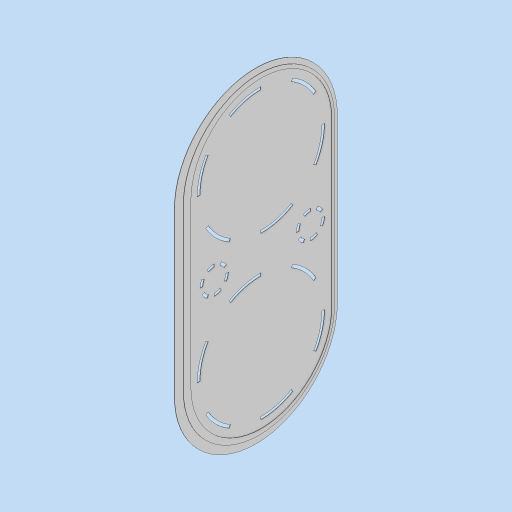
# Autodesk Inventor part: Sticker4
Saved by Autodesk Inventor 2024 (Build 280153000, 153)
## iProperties
Created: 2025-01-25
Part Number: Sticker4
Material: Generic
Document SubType Name: Modeling
Designer: Dmitry
Density: 1 g/cm^3
Appearance: Default
Author: Dmitry
Autodesk Inventor part; units mm, degrees
(part 1 of 2)
ref_plane "YZ Plane" through (0, 0, 0) normal (1, 0, 0) x (0, 1, 0)
ref_plane "XZ Plane" through (0, 0, 0) normal (0, 1, 0) x (-1, 0, 0)
ref_plane "XY Plane" through (0, 0, 0) normal (0, 0, 1) x (1, 0, 0)
sketch "Sketch1" plane through (0, 0, 0) normal (1, 0, 0) x (0, 1, 0)
  line L0 (-65.4167, -24.9139) -> (-65.4167, -26.1387)
  line L1 (-65.4167, -26.1387) -> (-65.6677, -29.8166)
  line L2 (-65.6677, -29.8166) -> (-66.4035, -34.5779)
  line L3 (-66.4035, -34.5779) -> (-67.5981, -39.175)
  line L4 (-67.5981, -39.175) -> (-69.2298, -43.5806)
  line L5 (-69.2298, -43.5806) -> (-71.2719, -47.7739)
  line L6 (-71.2719, -47.7739) -> (-73.7014, -51.7274)
  line L7 (-73.7014, -51.7274) -> (-76.4934, -55.4193)
  line L8 (-76.4934, -55.4193) -> (-79.6242, -58.8257)
  line L9 (-79.6242, -58.8257) -> (-83.0679, -61.921)
  line L10 (-83.0679, -61.921) -> (-86.8025, -64.6824)
  line L11 (-86.8025, -64.6824) -> (-90.8017, -67.0845)
  line L12 (-90.8017, -67.0845) -> (-95.0417, -69.1031)
  line L13 (-95.0417, -69.1031) -> (-99.4984, -70.717)
  line L14 (-99.4984, -70.717) -> (-104.1466, -71.8978)
  line L15 (-104.1466, -71.8978) -> (-108.9627, -72.6255)
  line L16 (-108.9627, -72.6255) -> (-112.682, -72.8737)
  line L17 (-112.682, -72.8737) -> (-113.9211, -72.8737)
  line L18 (-113.9211, -72.8737) -> (-115.1613, -72.8737)
  line L19 (-115.1613, -72.8737) -> (-118.8804, -72.6255)
  line L20 (-118.8804, -72.6255) -> (-123.6968, -71.8978)
  line L21 (-123.6968, -71.8978) -> (-128.345, -70.717)
  line L22 (-128.345, -70.717) -> (-132.8014, -69.1031)
  line L23 (-132.8014, -69.1031) -> (-137.0417, -67.0845)
  line L24 (-137.0417, -67.0845) -> (-141.0406, -64.6824)
  line L25 (-141.0406, -64.6824) -> (-144.7739, -61.921)
  line L26 (-144.7739, -61.921) -> (-148.2189, -58.8257)
  line L27 (-148.2189, -58.8257) -> (-151.3485, -55.4193)
  line L28 (-151.3485, -55.4193) -> (-154.1404, -51.7274)
  line L29 (-154.1404, -51.7274) -> (-156.5697, -47.7739)
  line L30 (-156.5697, -47.7739) -> (-158.6134, -43.5806)
  line L31 (-158.6134, -43.5806) -> (-160.2435, -39.175)
  line L32 (-160.2435, -39.175) -> (-161.4384, -34.5779)
  line L33 (-161.4384, -34.5779) -> (-162.1742, -29.8166)
  line L34 (-162.1742, -29.8166) -> (-162.4236, -26.1387)
  line L35 (-162.4236, -26.1387) -> (-162.4236, -24.9139)
  line L36 (-162.4236, -24.9139) -> (-162.4236, -23.6871)
  line L37 (-162.4236, -23.6871) -> (-162.1742, -20.0092)
  line L38 (-162.1742, -20.0092) -> (-161.4384, -15.2482)
  line L39 (-161.4384, -15.2482) -> (-160.2435, -10.6511)
  line L40 (-160.2435, -10.6511) -> (-158.6134, -6.2454)
  line L41 (-158.6134, -6.2454) -> (-156.5697, -2.0521)
  line L42 (-156.5697, -2.0521) -> (-154.1404, 1.9016)
  line L43 (-154.1404, 1.9016) -> (-151.3485, 5.5933)
  line L44 (-151.3485, 5.5933) -> (-148.2189, 8.9997)
  line L45 (-148.2189, 8.9997) -> (-144.7739, 12.0952)
  line L46 (-144.7739, 12.0952) -> (-141.0406, 14.8566)
  line L47 (-141.0406, 14.8566) -> (-137.0417, 17.2582)
  line L48 (-137.0417, 17.2582) -> (-132.8014, 19.2773)
  line L49 (-132.8014, 19.2773) -> (-128.345, 20.8909)
  line L50 (-128.345, 20.8909) -> (-123.6968, 22.072)
  line L51 (-123.6968, 22.072) -> (-118.8804, 22.7995)
  line L52 (-118.8804, 22.7995) -> (-115.1613, 23.0464)
  line L53 (-115.1613, 23.0464) -> (-113.9211, 23.0464)
  line L54 (-113.9211, 23.0464) -> (-112.682, 23.0464)
  line L55 (-112.682, 23.0464) -> (-108.9627, 22.7995)
  line L56 (-108.9627, 22.7995) -> (-104.1466, 22.072)
  line L57 (-104.1466, 22.072) -> (-99.4984, 20.8909)
  line L58 (-99.4984, 20.8909) -> (-95.0417, 19.2773)
  line L59 (-95.0417, 19.2773) -> (-90.8017, 17.2582)
  line L60 (-90.8017, 17.2582) -> (-86.8025, 14.8566)
  line L61 (-86.8025, 14.8566) -> (-83.0679, 12.0952)
  line L62 (-83.0679, 12.0952) -> (-79.6242, 8.9997)
  line L63 (-79.6242, 8.9997) -> (-76.4934, 5.5933)
  line L64 (-76.4934, 5.5933) -> (-73.7014, 1.9016)
  line L65 (-73.7014, 1.9016) -> (-71.2719, -2.0521)
  line L66 (-71.2719, -2.0521) -> (-69.2298, -6.2454)
  line L67 (-69.2298, -6.2454) -> (-67.5981, -10.6511)
  line L68 (-67.5981, -10.6511) -> (-66.4035, -15.2482)
  line L69 (-66.4035, -15.2482) -> (-65.6677, -20.0092)
  line L70 (-65.6677, -20.0092) -> (-65.4167, -23.6871)
  line L71 (-65.4167, -23.6871) -> (-65.4167, -24.9139)
  line L72 (53.0283, -25.7214) -> (53.0283, -26.9462)
  line L73 (53.0283, -26.9462) -> (52.7769, -30.6243)
  line L74 (52.7769, -30.6243) -> (52.0428, -35.3853)
  line L75 (52.0428, -35.3853) -> (50.8465, -39.9825)
  line L76 (50.8465, -39.9825) -> (49.2158, -44.3881)
  line L77 (49.2158, -44.3881) -> (47.1736, -48.5804)
  line L78 (47.1736, -48.5804) -> (44.7428, -52.5349)
  line L79 (44.7428, -52.5349) -> (41.9514, -56.2268)
  line L80 (41.9514, -56.2268) -> (38.8221, -59.6322)
  line L81 (38.8221, -59.6322) -> (35.3779, -62.7284)
  line L82 (35.3779, -62.7284) -> (31.6441, -65.4886)
  line L83 (31.6441, -65.4886) -> (27.6461, -67.8907)
  line L84 (27.6461, -67.8907) -> (23.4043, -69.9105)
  line L85 (23.4043, -69.9105) -> (18.9491, -71.5232)
  line L86 (18.9491, -71.5232) -> (14.3009, -72.704)
  line L87 (14.3009, -72.704) -> (9.4851, -73.4317)
  line L88 (9.4851, -73.4317) -> (5.764, -73.6796)
  line L89 (5.764, -73.6796) -> (4.5245, -73.6796)
  line L90 (4.5245, -73.6796) -> (3.285, -73.6796)
  line L91 (3.285, -73.6796) -> (-0.4336, -73.4317)
  line L92 (-0.4336, -73.4317) -> (-5.2494, -72.704)
  line L93 (-5.2494, -72.704) -> (-9.8976, -71.5232)
  line L94 (-9.8976, -71.5232) -> (-14.3553, -69.9105)
  line L95 (-14.3553, -69.9105) -> (-18.5946, -67.8907)
  line L96 (-18.5946, -67.8907) -> (-22.5941, -65.4886)
  line L97 (-22.5941, -65.4886) -> (-26.3287, -62.7284)
  line L98 (-26.3287, -62.7284) -> (-29.7726, -59.6322)
  line L99 (-29.7726, -59.6322) -> (-32.9034, -56.2268)
  line L100 (-32.9034, -56.2268) -> (-35.6954, -52.5349)
  line L101 (-35.6954, -52.5349) -> (-38.1244, -48.5804)
  line L102 (-38.1244, -48.5804) -> (-40.1668, -44.3881)
  line L103 (-40.1668, -44.3881) -> (-41.7983, -39.9825)
  line L104 (-41.7983, -39.9825) -> (-42.9931, -35.3853)
  line L105 (-42.9931, -35.3853) -> (-43.7292, -30.6243)
  line L106 (-43.7292, -30.6243) -> (-43.9786, -26.9462)
  line L107 (-43.9786, -26.9462) -> (-43.9786, -25.7214)
  line L108 (-43.9786, -25.7214) -> (-43.9786, -24.4948)
  line L109 (-43.9786, -24.4948) -> (-43.7292, -20.8166)
  line L110 (-43.7292, -20.8166) -> (-42.9931, -16.0557)
  line L111 (-42.9931, -16.0557) -> (-41.7983, -11.4585)
  line L112 (-41.7983, -11.4585) -> (-40.1668, -7.0531)
  line L113 (-40.1668, -7.0531) -> (-38.1244, -2.8596)
  line L114 (-38.1244, -2.8596) -> (-35.6954, 1.0939)
  line L115 (-35.6954, 1.0939) -> (-32.9034, 4.7858)
  line L116 (-32.9034, 4.7858) -> (-29.7726, 8.1922)
  line L117 (-29.7726, 8.1922) -> (-26.3287, 11.2874)
  line L118 (-26.3287, 11.2874) -> (-22.5941, 14.0492)
  line L119 (-22.5941, 14.0492) -> (-18.5946, 16.4507)
  line L120 (-18.5946, 16.4507) -> (-14.3553, 18.4698)
  line L121 (-14.3553, 18.4698) -> (-9.8976, 20.0835)
  line L122 (-9.8976, 20.0835) -> (-5.2494, 21.2646)
  line L123 (-5.2494, 21.2646) -> (-0.4336, 21.9918)
  line L124 (-0.4336, 21.9918) -> (3.285, 22.2389)
  line L125 (3.285, 22.2389) -> (4.5245, 22.2389)
  line L126 (4.5245, 22.2389) -> (5.764, 22.2389)
  line L127 (5.764, 22.2389) -> (9.4851, 21.9918)
  line L128 (9.4851, 21.9918) -> (14.3009, 21.2646)
  line L129 (14.3009, 21.2646) -> (18.9491, 20.0835)
  line L130 (18.9491, 20.0835) -> (23.4043, 18.4698)
  line L131 (23.4043, 18.4698) -> (27.6461, 16.4507)
  line L132 (27.6461, 16.4507) -> (31.6441, 14.0492)
  line L133 (31.6441, 14.0492) -> (35.3779, 11.2874)
  line L134 (35.3779, 11.2874) -> (38.8221, 8.1922)
  line L135 (38.8221, 8.1922) -> (41.9514, 4.7858)
  line L136 (41.9514, 4.7858) -> (44.7428, 1.0939)
  line L137 (44.7428, 1.0939) -> (47.1736, -2.8596)
  line L138 (47.1736, -2.8596) -> (49.2158, -7.0531)
  line L139 (49.2158, -7.0531) -> (50.8465, -11.4585)
  line L140 (50.8465, -11.4585) -> (52.0428, -16.0557)
  line L141 (52.0428, -16.0557) -> (52.7769, -20.8166)
  line L142 (52.7769, -20.8166) -> (53.0283, -24.4948)
  line L143 (53.0283, -24.4948) -> (53.0283, -25.7214)
  line L144 (-44.6979, 12.3512) -> (-44.6979, 11.8539)
  line L145 (-44.6979, 11.8539) -> (-44.9016, 10.3586)
  line L146 (-44.9016, 10.3586) -> (-45.4848, 8.5023)
  line L147 (-45.4848, 8.5023) -> (-46.4066, 6.8224)
  line L148 (-46.4066, 6.8224) -> (-47.6276, 5.3591)
  line L149 (-47.6276, 5.3591) -> (-49.1076, 4.1518)
  line L150 (-49.1076, 4.1518) -> (-50.8054, 3.2397)
  line L151 (-50.8054, 3.2397) -> (-52.6822, 2.6636)
  line L152 (-52.6822, 2.6636) -> (-54.194, 2.4625)
  line L153 (-54.194, 2.4625) -> (-54.6969, 2.4625)
  line L154 (-54.6969, 2.4625) -> (-55.2013, 2.4625)
  line L155 (-55.2013, 2.4625) -> (-56.7131, 2.6636)
  line L156 (-56.7131, 2.6636) -> (-58.59, 3.2397)
  line L157 (-58.59, 3.2397) -> (-60.2892, 4.1518)
  line L158 (-60.2892, 4.1518) -> (-61.769, 5.3591)
  line L159 (-61.769, 5.3591) -> (-62.99, 6.8224)
  line L160 (-62.99, 6.8224) -> (-63.9118, 8.5023)
  line L161 (-63.9118, 8.5023) -> (-64.4947, 10.3586)
  line L162 (-64.4947, 10.3586) -> (-64.6976, 11.8539)
  line L163 (-64.6976, 11.8539) -> (-64.6976, 12.3512)
  line L164 (-64.6976, 12.3512) -> (-64.6976, 12.85)
  line L165 (-64.6976, 12.85) -> (-64.4947, 14.3453)
  line L166 (-64.4947, 14.3453) -> (-63.9118, 16.2)
  line L167 (-63.9118, 16.2) -> (-62.99, 17.8798)
  line L168 (-62.99, 17.8798) -> (-61.769, 19.3436)
  line L169 (-61.769, 19.3436) -> (-60.2892, 20.5503)
  line L170 (-60.2892, 20.5503) -> (-58.59, 21.4627)
  line L171 (-58.59, 21.4627) -> (-56.7131, 22.0387)
  line L172 (-56.7131, 22.0387) -> (-55.2013, 22.2389)
  line L173 (-55.2013, 22.2389) -> (-54.6969, 22.2389)
  line L174 (-54.6969, 22.2389) -> (-54.194, 22.2389)
  line L175 (-54.194, 22.2389) -> (-52.6822, 22.0387)
  line L176 (-52.6822, 22.0387) -> (-50.8054, 21.4627)
  line L177 (-50.8054, 21.4627) -> (-49.1076, 20.5503)
  line L178 (-49.1076, 20.5503) -> (-47.6276, 19.3436)
  line L179 (-47.6276, 19.3436) -> (-46.4066, 17.8798)
  line L180 (-46.4066, 17.8798) -> (-45.4848, 16.2)
  line L181 (-45.4848, 16.2) -> (-44.9016, 14.3453)
  line L182 (-44.9016, 14.3453) -> (-44.6979, 12.85)
  line L183 (-44.6979, 12.85) -> (-44.6979, 12.3512)
  line L184 (-44.3009, -63.7924) -> (-44.3009, -64.2898)
  line L185 (-44.3009, -64.2898) -> (-44.5049, -65.7848)
  line L186 (-44.5049, -65.7848) -> (-45.0881, -67.6398)
  line L187 (-45.0881, -67.6398) -> (-46.0098, -69.3197)
  line L188 (-46.0098, -69.3197) -> (-47.2308, -70.783)
  line L189 (-47.2308, -70.783) -> (-48.7106, -71.9903)
  line L190 (-48.7106, -71.9903) -> (-50.4086, -72.9026)
  line L191 (-50.4086, -72.9026) -> (-52.2854, -73.4787)
  line L192 (-52.2854, -73.4787) -> (-53.797, -73.6796)
  line L193 (-53.797, -73.6796) -> (-54.3001, -73.6796)
  line L194 (-54.3001, -73.6796) -> (-54.8046, -73.6796)
  line L195 (-54.8046, -73.6796) -> (-56.3161, -73.4787)
  line L196 (-56.3161, -73.4787) -> (-58.193, -72.9026)
  line L197 (-58.193, -72.9026) -> (-59.8922, -71.9903)
  line L198 (-59.8922, -71.9903) -> (-61.3723, -70.783)
  line L199 (-61.3723, -70.783) -> (-62.5932, -69.3197)
  line L200 (-62.5932, -69.3197) -> (-63.515, -67.6398)
  line L201 (-63.515, -67.6398) -> (-64.0977, -65.7848)
  line L202 (-64.0977, -65.7848) -> (-64.3006, -64.2898)
  line L203 (-64.3006, -64.2898) -> (-64.3006, -63.7924)
  line L204 (-64.3006, -63.7924) -> (-64.3006, -63.2936)
  line L205 (-64.3006, -63.2936) -> (-64.0977, -61.7983)
  line L206 (-64.0977, -61.7983) -> (-63.515, -59.9433)
  line L207 (-63.515, -59.9433) -> (-62.5932, -58.2636)
  line L208 (-62.5932, -58.2636) -> (-61.3723, -56.8001)
  line L209 (-61.3723, -56.8001) -> (-59.8922, -55.5928)
  line L210 (-59.8922, -55.5928) -> (-58.193, -54.6804)
  line L211 (-58.193, -54.6804) -> (-56.3161, -54.1049)
  line L212 (-56.3161, -54.1049) -> (-54.8046, -53.9047)
  line L213 (-54.8046, -53.9047) -> (-54.3001, -53.9047)
  line L214 (-54.3001, -53.9047) -> (-53.797, -53.9047)
  line L215 (-53.797, -53.9047) -> (-52.2854, -54.1049)
  line L216 (-52.2854, -54.1049) -> (-50.4086, -54.6804)
  line L217 (-50.4086, -54.6804) -> (-48.7106, -55.5928)
  line L218 (-48.7106, -55.5928) -> (-47.2308, -56.8001)
  line L219 (-47.2308, -56.8001) -> (-46.0098, -58.2636)
  line L220 (-46.0098, -58.2636) -> (-45.0881, -59.9433)
  line L221 (-45.0881, -59.9433) -> (-44.5049, -61.7983)
  line L222 (-44.5049, -61.7983) -> (-44.3009, -63.2936)
  line L223 (-44.3009, -63.2936) -> (-44.3009, -63.7924)
  line L224 (2.8024, -74.4653) -> (-112.1984, -74.4653)
  line L225 (-112.1984, -74.4653) -> (-113.663, -74.4653)
  line L226 (-113.663, -74.4653) -> (-118.0564, -74.1663)
  line L227 (-118.0564, -74.1663) -> (-123.7491, -73.291)
  line L228 (-123.7491, -73.291) -> (-129.2487, -71.8676)
  line L229 (-129.2487, -71.8676) -> (-134.5253, -69.9273)
  line L230 (-134.5253, -69.9273) -> (-139.5481, -67.498)
  line L231 (-139.5481, -67.498) -> (-144.2901, -64.6095)
  line L232 (-144.2901, -64.6095) -> (-148.7193, -61.2913)
  line L233 (-148.7193, -61.2913) -> (-152.8077, -57.5732)
  line L234 (-152.8077, -57.5732) -> (-156.5255, -53.4846)
  line L235 (-156.5255, -53.4846) -> (-159.8443, -49.0556)
  line L236 (-159.8443, -49.0556) -> (-162.7322, -44.3137)
  line L237 (-162.7322, -44.3137) -> (-165.162, -39.2906)
  line L238 (-165.162, -39.2906) -> (-167.1023, -34.014)
  line L239 (-167.1023, -34.014) -> (-168.5257, -28.5146)
  line L240 (-168.5257, -28.5146) -> (-169.401, -22.822)
  line L241 (-169.401, -22.822) -> (-169.6982, -18.4288)
  line L242 (-169.6982, -18.4288) -> (-169.6982, -16.965)
  line L243 (-169.6982, -16.965) -> (-169.6982, -15.5004)
  line L244 (-169.6982, -15.5004) -> (-169.401, -11.1072)
  line L245 (-169.401, -11.1072) -> (-168.5257, -5.4131)
  line L246 (-168.5257, -5.4131) -> (-167.1023, 0.0855)
  line L247 (-167.1023, 0.0855) -> (-165.162, 5.3619)
  line L248 (-165.162, 5.3619) -> (-162.7322, 10.3862)
  line L249 (-162.7322, 10.3862) -> (-159.8443, 15.1264)
  line L250 (-159.8443, 15.1264) -> (-156.5255, 19.5569)
  line L251 (-156.5255, 19.5569) -> (-152.8077, 23.6458)
  line L252 (-152.8077, 23.6458) -> (-148.7193, 27.3636)
  line L253 (-148.7193, 27.3636) -> (-144.2901, 30.6803)
  line L254 (-144.2901, 30.6803) -> (-139.5481, 33.5691)
  line L255 (-139.5481, 33.5691) -> (-134.5253, 35.9981)
  line L256 (-134.5253, 35.9981) -> (-129.2487, 37.9384)
  line L257 (-129.2487, 37.9384) -> (-123.7491, 39.3623)
  line L258 (-123.7491, 39.3623) -> (-118.0564, 40.2371)
  line L259 (-118.0564, 40.2371) -> (-113.663, 40.535)
  line L260 (-113.663, 40.535) -> (-112.1984, 40.535)
  line L261 (-112.1984, 40.535) -> (2.8024, 40.535)
  line L262 (2.8024, 40.535) -> (4.2654, 40.535)
  line L263 (4.2654, 40.535) -> (8.6596, 40.2371)
  line L264 (8.6596, 40.2371) -> (14.3517, 39.3623)
  line L265 (14.3517, 39.3623) -> (19.8508, 37.9384)
  line L266 (19.8508, 37.9384) -> (25.1264, 35.9981)
  line L267 (25.1264, 35.9981) -> (30.1505, 33.5691)
  line L268 (30.1505, 33.5691) -> (34.8927, 30.6803)
  line L269 (34.8927, 30.6803) -> (39.3225, 27.3636)
  line L270 (39.3225, 27.3636) -> (43.4119, 23.6458)
  line L271 (43.4119, 23.6458) -> (47.1279, 19.5569)
  line L272 (47.1279, 19.5569) -> (50.4451, 15.1264)
  line L273 (50.4451, 15.1264) -> (53.3331, 10.3862)
  line L274 (53.3331, 10.3862) -> (55.7639, 5.3619)
  line L275 (55.7639, 5.3619) -> (57.7045, 0.0855)
  line L276 (57.7045, 0.0855) -> (59.1269, -5.4131)
  line L277 (59.1269, -5.4131) -> (60.0032, -11.1072)
  line L278 (60.0032, -11.1072) -> (60.3003, -15.5004)
  line L279 (60.3003, -15.5004) -> (60.3003, -16.965)
  line L280 (60.3003, -16.965) -> (60.3003, -18.4288)
  line L281 (60.3003, -18.4288) -> (60.0032, -22.822)
  line L282 (60.0032, -22.822) -> (59.1269, -28.5146)
  line L283 (59.1269, -28.5146) -> (57.7045, -34.014)
  line L284 (57.7045, -34.014) -> (55.7639, -39.2906)
  line L285 (55.7639, -39.2906) -> (53.3331, -44.3137)
  line L286 (53.3331, -44.3137) -> (50.4451, -49.0556)
  line L287 (50.4451, -49.0556) -> (47.1279, -53.4846)
  line L288 (47.1279, -53.4846) -> (43.4119, -57.5732)
  line L289 (43.4119, -57.5732) -> (39.3225, -61.2913)
  line L290 (39.3225, -61.2913) -> (34.8927, -64.6095)
  line L291 (34.8927, -64.6095) -> (30.1505, -67.498)
  line L292 (30.1505, -67.498) -> (25.1264, -69.9273)
  line L293 (25.1264, -69.9273) -> (19.8508, -71.8676)
  line L294 (19.8508, -71.8676) -> (14.3517, -73.291)
  line L295 (14.3517, -73.291) -> (8.6596, -74.1663)
  line L296 (8.6596, -74.1663) -> (4.2654, -74.4653)
  line L297 (4.2654, -74.4653) -> (2.8024, -74.4653)
  line L298 (2.4518, -72.2478) -> (-111.8469, -72.2478)
  line L299 (-111.8469, -72.2478) -> (-113.2068, -72.2478)
  line L300 (-113.2068, -72.2478) -> (-117.2833, -71.971)
  line L301 (-117.2833, -71.971) -> (-122.5667, -71.1582)
  line L302 (-122.5667, -71.1582) -> (-127.6708, -69.8376)
  line L303 (-127.6708, -69.8376) -> (-132.5669, -68.0368)
  line L304 (-132.5669, -68.0368) -> (-137.2289, -65.782)
  line L305 (-137.2289, -65.782) -> (-141.6292, -63.1021)
  line L306 (-141.6292, -63.1021) -> (-145.7412, -60.022)
  line L307 (-145.7412, -60.022) -> (-149.5349, -56.5715)
  line L308 (-149.5349, -56.5715) -> (-152.9855, -52.7777)
  line L309 (-152.9855, -52.7777) -> (-156.0655, -48.6657)
  line L310 (-156.0655, -48.6657) -> (-158.7457, -44.2654)
  line L311 (-158.7457, -44.2654) -> (-161.0002, -39.6035)
  line L312 (-161.0002, -39.6035) -> (-162.8011, -34.7074)
  line L313 (-162.8011, -34.7074) -> (-164.1216, -29.6033)
  line L314 (-164.1216, -29.6033) -> (-164.9344, -24.3198)
  line L315 (-164.9344, -24.3198) -> (-165.2103, -20.2434)
  line L316 (-165.2103, -20.2434) -> (-165.2103, -18.885)
  line L317 (-165.2103, -18.885) -> (-165.2103, -17.5245)
  line L318 (-165.2103, -17.5245) -> (-164.9344, -13.4486)
  line L319 (-164.9344, -13.4486) -> (-164.1216, -8.1636)
  line L320 (-164.1216, -8.1636) -> (-162.8011, -3.0608)
  line L321 (-162.8011, -3.0608) -> (-161.0002, 1.8369)
  line L322 (-161.0002, 1.8369) -> (-158.7457, 6.4985)
  line L323 (-158.7457, 6.4985) -> (-156.0655, 10.8988)
  line L324 (-156.0655, 10.8988) -> (-152.9855, 15.0093)
  line L325 (-152.9855, 15.0093) -> (-149.5349, 18.8046)
  line L326 (-149.5349, 18.8046) -> (-145.7412, 22.2552)
  line L327 (-145.7412, 22.2552) -> (-141.6292, 25.3336)
  line L328 (-141.6292, 25.3336) -> (-137.2289, 28.0141)
  line L329 (-137.2289, 28.0141) -> (-132.5669, 30.2683)
  line L330 (-132.5669, 30.2683) -> (-127.6708, 32.0697)
  line L331 (-127.6708, 32.0697) -> (-122.5667, 33.3898)
  line L332 (-122.5667, 33.3898) -> (-117.2833, 34.2028)
  line L333 (-117.2833, 34.2028) -> (-113.2068, 34.4784)
  line L334 (-113.2068, 34.4784) -> (-111.8469, 34.4784)
  line L335 (-111.8469, 34.4784) -> (2.4518, 34.4784)
  line L336 (2.4518, 34.4784) -> (3.8107, 34.4784)
  line L337 (3.8107, 34.4784) -> (7.8874, 34.2028)
  line L338 (7.8874, 34.2028) -> (13.1706, 33.3898)
  line L339 (13.1706, 33.3898) -> (18.2735, 32.0697)
  line L340 (18.2735, 32.0697) -> (23.1706, 30.2683)
  line L341 (23.1706, 30.2683) -> (27.8315, 28.0141)
  line L342 (27.8315, 28.0141) -> (32.2333, 25.3336)
  line L343 (32.2333, 25.3336) -> (36.3456, 22.2552)
  line L344 (36.3456, 22.2552) -> (40.1378, 18.8046)
  line L345 (40.1378, 18.8046) -> (43.5897, 15.0093)
  line L346 (43.5897, 15.0093) -> (46.6682, 10.8988)
  line L347 (46.6682, 10.8988) -> (49.3504, 6.4985)
  line L348 (49.3504, 6.4985) -> (51.6034, 1.8369)
  line L349 (51.6034, 1.8369) -> (53.4042, -3.0608)
  line L350 (53.4042, -3.0608) -> (54.725, -8.1636)
  line L351 (54.725, -8.1636) -> (55.5378, -13.4486)
  line L352 (55.5378, -13.4486) -> (55.8147, -17.5245)
  line L353 (55.8147, -17.5245) -> (55.8147, -18.885)
  line L354 (55.8147, -18.885) -> (55.8147, -20.2434)
  line L355 (55.8147, -20.2434) -> (55.5378, -24.3198)
  line L356 (55.5378, -24.3198) -> (54.725, -29.6033)
  line L357 (54.725, -29.6033) -> (53.4042, -34.7074)
  line L358 (53.4042, -34.7074) -> (51.6034, -39.6035)
  line L359 (51.6034, -39.6035) -> (49.3504, -44.2654)
  line L360 (49.3504, -44.2654) -> (46.6682, -48.6657)
  line L361 (46.6682, -48.6657) -> (43.5897, -52.7777)
  line L362 (43.5897, -52.7777) -> (40.1378, -56.5715)
  line L363 (40.1378, -56.5715) -> (36.3456, -60.022)
  line L364 (36.3456, -60.022) -> (32.2333, -63.1021)
  line L365 (32.2333, -63.1021) -> (27.8315, -65.782)
  line L366 (27.8315, -65.782) -> (23.1706, -68.0368)
  line L367 (23.1706, -68.0368) -> (18.2735, -69.8376)
  line L368 (18.2735, -69.8376) -> (13.1706, -71.1582)
  line L369 (13.1706, -71.1582) -> (7.8874, -71.971)
  line L370 (7.8874, -71.971) -> (3.8107, -72.2478)
  line L371 (3.8107, -72.2478) -> (2.4518, -72.2478)
  line L372 (2.8049, -70.4084) -> (-112.2012, -70.4084)
  line L373 (-112.2012, -70.4084) -> (-113.4705, -70.4084)
  line L374 (-113.4705, -70.4084) -> (-117.2779, -70.149)
  line L375 (-117.2779, -70.149) -> (-122.2126, -69.3898)
  line L376 (-122.2126, -69.3898) -> (-126.9779, -68.1579)
  line L377 (-126.9779, -68.1579) -> (-131.5515, -66.4752)
  line L378 (-131.5515, -66.4752) -> (-135.9048, -64.3695)
  line L379 (-135.9048, -64.3695) -> (-140.0142, -61.8674)
  line L380 (-140.0142, -61.8674) -> (-143.8534, -58.9911)
  line L381 (-143.8534, -58.9911) -> (-147.3965, -55.7691)
  line L382 (-147.3965, -55.7691) -> (-150.6195, -52.2253)
  line L383 (-150.6195, -52.2253) -> (-153.4943, -48.3858)
  line L384 (-153.4943, -48.3858) -> (-155.9979, -44.2763)
  line L385 (-155.9979, -44.2763) -> (-158.1036, -39.923)
  line L386 (-158.1036, -39.923) -> (-159.7863, -35.351)
  line L387 (-159.7863, -35.351) -> (-161.0182, -30.5845)
  line L388 (-161.0182, -30.5845) -> (-161.7775, -25.6498)
  line L389 (-161.7775, -25.6498) -> (-162.0353, -21.8423)
  line L390 (-162.0353, -21.8423) -> (-162.0353, -20.5743)
  line L391 (-162.0353, -20.5743) -> (-162.0353, -19.3051)
  line L392 (-162.0353, -19.3051) -> (-161.7775, -15.4974)
  line L393 (-161.7775, -15.4974) -> (-161.0182, -10.5629)
  line L394 (-161.0182, -10.5629) -> (-159.7863, -5.7976)
  line L395 (-159.7863, -5.7976) -> (-158.1036, -1.2251)
  line L396 (-158.1036, -1.2251) -> (-155.9979, 3.1295)
  line L397 (-155.9979, 3.1295) -> (-153.4943, 7.2387)
  line L398 (-153.4943, 7.2387) -> (-150.6195, 11.0779)
  line L399 (-150.6195, 11.0779) -> (-147.3965, 14.6209)
  line L400 (-147.3965, 14.6209) -> (-143.8534, 17.8429)
  line L401 (-143.8534, 17.8429) -> (-140.0142, 20.7187)
  line L402 (-140.0142, 20.7187) -> (-135.9048, 23.2214)
  line L403 (-135.9048, 23.2214) -> (-131.5515, 25.3268)
  line L404 (-131.5515, 25.3268) -> (-126.9779, 27.0095)
  line L405 (-126.9779, 27.0095) -> (-122.2126, 28.2414)
  line L406 (-122.2126, 28.2414) -> (-117.2779, 29.0009)
  line L407 (-117.2779, 29.0009) -> (-113.4705, 29.2584)
  line L408 (-113.4705, 29.2584) -> (-112.2012, 29.2584)
  line L409 (-112.2012, 29.2584) -> (2.8049, 29.2584)
  line L410 (2.8049, 29.2584) -> (4.0724, 29.2584)
  line L411 (4.0724, 29.2584) -> (7.8798, 29.0009)
  line L412 (7.8798, 29.0009) -> (12.815, 28.2414)
  line L413 (12.815, 28.2414) -> (17.5801, 27.0095)
  line L414 (17.5801, 27.0095) -> (22.1546, 25.3268)
  line L415 (22.1546, 25.3268) -> (26.5056, 23.2214)
  line L416 (26.5056, 23.2214) -> (30.6154, 20.7187)
  line L417 (30.6154, 20.7187) -> (34.4558, 17.8429)
  line L418 (34.4558, 17.8429) -> (37.9991, 14.6209)
  line L419 (37.9991, 14.6209) -> (41.2224, 11.0779)
  line L420 (41.2224, 11.0779) -> (44.0977, 7.2387)
  line L421 (44.0977, 7.2387) -> (46.5996, 3.1295)
  line L422 (46.5996, 3.1295) -> (48.7052, -1.2251)
  line L423 (48.7052, -1.2251) -> (50.3893, -5.7976)
  line L424 (50.3893, -5.7976) -> (51.6212, -10.5629)
  line L425 (51.6212, -10.5629) -> (52.3781, -15.4974)
  line L426 (52.3781, -15.4974) -> (52.6397, -19.3051)
  line L427 (52.6397, -19.3051) -> (52.6397, -20.5743)
  line L428 (52.6397, -20.5743) -> (52.6397, -21.8423)
  line L429 (52.6397, -21.8423) -> (52.3781, -25.6498)
  line L430 (52.3781, -25.6498) -> (51.6212, -30.5845)
  line L431 (51.6212, -30.5845) -> (50.3893, -35.351)
  line L432 (50.3893, -35.351) -> (48.7052, -39.923)
  line L433 (48.7052, -39.923) -> (46.5996, -44.2763)
  line L434 (46.5996, -44.2763) -> (44.0977, -48.3858)
  line L435 (44.0977, -48.3858) -> (41.2224, -52.2253)
  line L436 (41.2224, -52.2253) -> (37.9991, -55.7691)
  line L437 (37.9991, -55.7691) -> (34.4558, -58.9911)
  line L438 (34.4558, -58.9911) -> (30.6154, -61.8674)
  line L439 (30.6154, -61.8674) -> (26.5056, -64.3695)
  line L440 (26.5056, -64.3695) -> (22.1546, -66.4752)
  line L441 (22.1546, -66.4752) -> (17.5801, -68.1579)
  line L442 (17.5801, -68.1579) -> (12.815, -69.3898)
  line L443 (12.815, -69.3898) -> (7.8798, -70.149)
  line L444 (7.8798, -70.149) -> (4.0724, -70.4084)
  line L445 (4.0724, -70.4084) -> (2.8049, -70.4084)
  line L446 (2.8049, -70.4071) -> (-112.2012, -70.4071)
  line L447 (-112.2012, -70.4071) -> (-113.4705, -70.4071)
  line L448 (-113.4705, -70.4071) -> (-117.2779, -70.1478)
  line L449 (-117.2779, -70.1478) -> (-122.2126, -69.3886)
  line L450 (-122.2126, -69.3886) -> (-126.9779, -68.1567)
  line L451 (-126.9779, -68.1567) -> (-131.5502, -66.4739)
  line L452 (-131.5502, -66.4739) -> (-135.9048, -64.3682)
  line L453 (-135.9048, -64.3682) -> (-140.0142, -61.8658)
  line L454 (-140.0142, -61.8658) -> (-143.8534, -58.9898)
  line L455 (-143.8534, -58.9898) -> (-147.3965, -55.7681)
  line L456 (-147.3965, -55.7681) -> (-150.618, -52.2253)
  line L457 (-150.618, -52.2253) -> (-153.4943, -48.3858)
  line L458 (-153.4943, -48.3858) -> (-155.9964, -44.2763)
  line L459 (-155.9964, -44.2763) -> (-158.1021, -39.922)
  line L460 (-158.1021, -39.922) -> (-159.7848, -35.3498)
  line L461 (-159.7848, -35.3498) -> (-161.0167, -30.5845)
  line L462 (-161.0167, -30.5845) -> (-161.7759, -25.6498)
  line L463 (-161.7759, -25.6498) -> (-162.0337, -21.8423)
  line L464 (-162.0337, -21.8423) -> (-162.0337, -20.5743)
  line L465 (-162.0337, -20.5743) -> (-162.0337, -19.3051)
  line L466 (-162.0337, -19.3051) -> (-161.7759, -15.4974)
  line L467 (-161.7759, -15.4974) -> (-161.0167, -10.5629)
  line L468 (-161.0167, -10.5629) -> (-159.7848, -5.7961)
  line L469 (-159.7848, -5.7961) -> (-158.1021, -1.2238)
  line L470 (-158.1021, -1.2238) -> (-155.9964, 3.1295)
  line L471 (-155.9964, 3.1295) -> (-153.4943, 7.2387)
  line L472 (-153.4943, 7.2387) -> (-150.618, 11.0779)
  line L473 (-150.618, 11.0779) -> (-147.3965, 14.6225)
  line L474 (-147.3965, 14.6225) -> (-143.8534, 17.8442)
  line L475 (-143.8534, 17.8442) -> (-140.0142, 20.72)
  line L476 (-140.0142, 20.72) -> (-135.9048, 23.2226)
  line L477 (-135.9048, 23.2226) -> (-131.5502, 25.328)
  line L478 (-131.5502, 25.328) -> (-126.9779, 27.0108)
  line L479 (-126.9779, 27.0108) -> (-122.2126, 28.2427)
  line L480 (-122.2126, 28.2427) -> (-117.2779, 29.0019)
  line L481 (-117.2779, 29.0019) -> (-113.4705, 29.2597)
  line L482 (-113.4705, 29.2597) -> (-112.2012, 29.2597)
  line L483 (-112.2012, 29.2597) -> (2.8049, 29.2597)
  line L484 (2.8049, 29.2597) -> (4.0724, 29.2597)
  line L485 (4.0724, 29.2597) -> (7.8798, 29.0019)
  line L486 (7.8798, 29.0019) -> (12.815, 28.2427)
  line L487 (12.815, 28.2427) -> (17.5801, 27.0108)
  line L488 (17.5801, 27.0108) -> (22.1546, 25.328)
  line L489 (22.1546, 25.328) -> (26.5056, 23.2226)
  line L490 (26.5056, 23.2226) -> (30.6154, 20.72)
  line L491 (30.6154, 20.72) -> (34.4558, 17.8442)
  line L492 (34.4558, 17.8442) -> (37.9991, 14.6225)
  line L493 (37.9991, 14.6225) -> (41.2224, 11.0779)
  line L494 (41.2224, 11.0779) -> (44.0977, 7.2387)
  line L495 (44.0977, 7.2387) -> (46.5996, 3.1295)
  line L496 (46.5996, 3.1295) -> (48.7052, -1.2238)
  line L497 (48.7052, -1.2238) -> (50.3893, -5.7961)
  line L498 (50.3893, -5.7961) -> (51.6212, -10.5629)
  line L499 (51.6212, -10.5629) -> (52.3781, -15.4974)
  line L500 (52.3781, -15.4974) -> (52.6397, -19.3051)
  line L501 (52.6397, -19.3051) -> (52.6397, -20.5743)
  line L502 (52.6397, -20.5743) -> (52.6397, -21.8423)
  line L503 (52.6397, -21.8423) -> (52.3781, -25.6498)
  line L504 (52.3781, -25.6498) -> (51.6212, -30.5845)
  line L505 (51.6212, -30.5845) -> (50.3893, -35.3498)
  line L506 (50.3893, -35.3498) -> (48.7052, -39.922)
  line L507 (48.7052, -39.922) -> (46.5996, -44.2763)
  line L508 (46.5996, -44.2763) -> (44.0977, -48.3858)
  line L509 (44.0977, -48.3858) -> (41.2224, -52.2253)
  line L510 (41.2224, -52.2253) -> (37.9991, -55.7681)
  line L511 (37.9991, -55.7681) -> (34.4558, -58.9898)
  line L512 (34.4558, -58.9898) -> (30.6154, -61.8658)
  line L513 (30.6154, -61.8658) -> (26.5056, -64.3682)
  line L514 (26.5056, -64.3682) -> (22.1546, -66.4739)
  line L515 (22.1546, -66.4739) -> (17.5801, -68.1567)
  line L516 (17.5801, -68.1567) -> (12.815, -69.3886)
  line L517 (12.815, -69.3886) -> (7.8798, -70.1478)
  line L518 (7.8798, -70.1478) -> (4.0724, -70.4071)
  line L519 (4.0724, -70.4071) -> (2.8049, -70.4071)
  line L520 (-64.9702, -20.187) -> (-64.9702, -21.361)
  line L521 (-64.9702, -21.361) -> (-65.2115, -24.886)
  line L522 (-65.2115, -24.886) -> (-65.9156, -29.4488)
  line L523 (-65.9156, -29.4488) -> (-67.0609, -33.8542)
  line L524 (-67.0609, -33.8542) -> (-68.6235, -38.0767)
  line L525 (-68.6235, -38.0767) -> (-70.5815, -42.0937)
  line L526 (-70.5815, -42.0937) -> (-72.9092, -45.8834)
  line L527 (-72.9092, -45.8834) -> (-75.5853, -49.4221)
  line L528 (-75.5853, -49.4221) -> (-78.5853, -52.6865)
  line L529 (-78.5853, -52.6865) -> (-81.8868, -55.652)
  line L530 (-81.8868, -55.652) -> (-85.4644, -58.2979)
  line L531 (-85.4644, -58.2979) -> (-89.2968, -60.6009)
  line L532 (-89.2968, -60.6009) -> (-93.3608, -62.5354)
  line L533 (-93.3608, -62.5354) -> (-97.631, -64.0817)
  line L534 (-97.631, -64.0817) -> (-102.0862, -65.2146)
  line L535 (-102.0862, -65.2146) -> (-106.7014, -65.9105)
  line L536 (-106.7014, -65.9105) -> (-110.265, -66.1485)
  line L537 (-110.265, -66.1485) -> (-111.4529, -66.1485)
  line L538 (-111.4529, -66.1485) -> (-112.6422, -66.1485)
  line L539 (-112.6422, -66.1485) -> (-116.2055, -65.9105)
  line L540 (-116.2055, -65.9105) -> (-120.8205, -65.2146)
  line L541 (-120.8205, -65.2146) -> (-125.2759, -64.0817)
  line L542 (-125.2759, -64.0817) -> (-129.5466, -62.5354)
  line L543 (-129.5466, -62.5354) -> (-133.6101, -60.6009)
  line L544 (-133.6101, -60.6009) -> (-137.4427, -58.2979)
  line L545 (-137.4427, -58.2979) -> (-141.0198, -55.652)
  line L546 (-141.0198, -55.652) -> (-144.3218, -52.6865)
  line L547 (-144.3218, -52.6865) -> (-147.3221, -49.4221)
  line L548 (-147.3221, -49.4221) -> (-149.9982, -45.8834)
  line L549 (-149.9982, -45.8834) -> (-152.3254, -42.0937)
  line L550 (-152.3254, -42.0937) -> (-154.2837, -38.0767)
  line L551 (-154.2837, -38.0767) -> (-155.8466, -33.8542)
  line L552 (-155.8466, -33.8542) -> (-156.9916, -29.4488)
  line L553 (-156.9916, -29.4488) -> (-157.6957, -24.886)
  line L554 (-157.6957, -24.886) -> (-157.9357, -21.361)
  line L555 (-157.9357, -21.361) -> (-157.9357, -20.187)
  line L556 (-157.9357, -20.187) -> (-157.9357, -19.0115)
  line L557 (-157.9357, -19.0115) -> (-157.6957, -15.4865)
  line L558 (-157.6957, -15.4865) -> (-156.9916, -10.9238)
  line L559 (-156.9916, -10.9238) -> (-155.8466, -6.5197)
  line L560 (-155.8466, -6.5197) -> (-154.2837, -2.2957)
  line L561 (-154.2837, -2.2957) -> (-152.3254, 1.7208)
  line L562 (-152.3254, 1.7208) -> (-149.9982, 5.5107)
  line L563 (-149.9982, 5.5107) -> (-147.3221, 9.0494)
  line L564 (-147.3221, 9.0494) -> (-144.3218, 12.3126)
  line L565 (-144.3218, 12.3126) -> (-141.0198, 15.2796)
  line L566 (-141.0198, 15.2796) -> (-137.4427, 17.9255)
  line L567 (-137.4427, 17.9255) -> (-133.6101, 20.2265)
  line L568 (-133.6101, 20.2265) -> (-129.5466, 22.163)
  line L569 (-129.5466, 22.163) -> (-125.2759, 23.7078)
  line L570 (-125.2759, 23.7078) -> (-120.8205, 24.8406)
  line L571 (-120.8205, 24.8406) -> (-116.2055, 25.5363)
  line L572 (-116.2055, 25.5363) -> (-112.6422, 25.7733)
  line L573 (-112.6422, 25.7733) -> (-111.4529, 25.7733)
  line L574 (-111.4529, 25.7733) -> (-110.265, 25.7733)
  line L575 (-110.265, 25.7733) -> (-106.7014, 25.5363)
  line L576 (-106.7014, 25.5363) -> (-102.0862, 24.8406)
  line L577 (-102.0862, 24.8406) -> (-97.631, 23.7078)
  line L578 (-97.631, 23.7078) -> (-93.3608, 22.163)
  line L579 (-93.3608, 22.163) -> (-89.2968, 20.2265)
  line L580 (-89.2968, 20.2265) -> (-85.4644, 17.9255)
  line L581 (-85.4644, 17.9255) -> (-81.8868, 15.2796)
  line L582 (-81.8868, 15.2796) -> (-78.5853, 12.3126)
  line L583 (-78.5853, 12.3126) -> (-75.5853, 9.0494)
  line L584 (-75.5853, 9.0494) -> (-72.9092, 5.5107)
  line L585 (-72.9092, 5.5107) -> (-70.5815, 1.7208)
  line L586 (-70.5815, 1.7208) -> (-68.6235, -2.2957)
  line L587 (-68.6235, -2.2957) -> (-67.0609, -6.5197)
  line L588 (-67.0609, -6.5197) -> (-65.9156, -10.9238)
  line L589 (-65.9156, -10.9238) -> (-65.2115, -15.4865)
  line L590 (-65.2115, -15.4865) -> (-64.9702, -19.0115)
  line L591 (-64.9702, -19.0115) -> (-64.9702, -20.187)
  line L592 (48.5401, -20.9614) -> (48.5401, -22.1357)
  line L593 (48.5401, -22.1357) -> (48.2988, -25.6607)
  line L594 (48.2988, -25.6607) -> (47.5953, -30.223)
  line L595 (47.5953, -30.223) -> (46.4497, -34.6276)
  line L596 (46.4497, -34.6276) -> (44.8876, -38.8511)
  line L597 (44.8876, -38.8511) -> (42.9293, -42.8682)
  line L598 (42.9293, -42.8682) -> (40.6026, -46.6576)
  line L599 (40.6026, -46.6576) -> (37.9255, -50.1968)
  line L600 (37.9255, -50.1968) -> (34.9257, -53.46)
  line L601 (34.9257, -53.46) -> (31.6237, -56.4267)
  line L602 (31.6237, -56.4267) -> (28.0449, -59.0726)
  line L603 (28.0449, -59.0726) -> (24.2146, -61.3738)
  line L604 (24.2146, -61.3738) -> (20.1506, -63.3098)
  line L605 (20.1506, -63.3098) -> (15.8783, -64.8547)
  line L606 (15.8783, -64.8547) -> (11.4231, -65.9875)
  line L607 (11.4231, -65.9875) -> (6.8079, -66.6835)
  line L608 (6.8079, -66.6835) -> (3.2443, -66.922)
  line L609 (3.2443, -66.922) -> (2.0581, -66.922)
  line L610 (2.0581, -66.922) -> (0.8694, -66.922)
  line L611 (0.8694, -66.922) -> (-2.6942, -66.6835)
  line L612 (-2.6942, -66.6835) -> (-7.3094, -65.9875)
  line L613 (-7.3094, -65.9875) -> (-11.7645, -64.8547)
  line L614 (-11.7645, -64.8547) -> (-16.0368, -63.3098)
  line L615 (-16.0368, -63.3098) -> (-20.1008, -61.3738)
  line L616 (-20.1008, -61.3738) -> (-23.9322, -59.0726)
  line L617 (-23.9322, -59.0726) -> (-27.5098, -56.4267)
  line L618 (-27.5098, -56.4267) -> (-30.8115, -53.46)
  line L619 (-30.8115, -53.46) -> (-33.8115, -50.1968)
  line L620 (-33.8115, -50.1968) -> (-36.4876, -46.6576)
  line L621 (-36.4876, -46.6576) -> (-38.8148, -42.8682)
  line L622 (-38.8148, -42.8682) -> (-40.7731, -38.8511)
  line L623 (-40.7731, -38.8511) -> (-42.336, -34.6276)
  line L624 (-42.336, -34.6276) -> (-43.481, -30.223)
  line L625 (-43.481, -30.223) -> (-44.1854, -25.6607)
  line L626 (-44.1854, -25.6607) -> (-44.4251, -22.1357)
  line L627 (-44.4251, -22.1357) -> (-44.4251, -20.9614)
  line L628 (-44.4251, -20.9614) -> (-44.4251, -19.7859)
  line L629 (-44.4251, -19.7859) -> (-44.1854, -16.2609)
  line L630 (-44.1854, -16.2609) -> (-43.481, -11.6983)
  line L631 (-43.481, -11.6983) -> (-42.336, -7.2927)
  line L632 (-42.336, -7.2927) -> (-40.7731, -3.0704)
  line L633 (-40.7731, -3.0704) -> (-38.8148, 0.9466)
  line L634 (-38.8148, 0.9466) -> (-36.4876, 4.736)
  line L635 (-36.4876, 4.736) -> (-33.8115, 8.2752)
  line L636 (-33.8115, 8.2752) -> (-30.8115, 11.5384)
  line L637 (-30.8115, 11.5384) -> (-27.5098, 14.5051)
  line L638 (-27.5098, 14.5051) -> (-23.9322, 17.151)
  line L639 (-23.9322, 17.151) -> (-20.1008, 19.4535)
  line L640 (-20.1008, 19.4535) -> (-16.0368, 21.3883)
  line L641 (-16.0368, 21.3883) -> (-11.7645, 22.9344)
  line L642 (-11.7645, 22.9344) -> (-7.3094, 24.0672)
  line L643 (-7.3094, 24.0672) -> (-2.6942, 24.7632)
  line L644 (-2.6942, 24.7632) -> (0.8694, 25.0004)
  line L645 (0.8694, 25.0004) -> (2.0581, 25.0004)
  line L646 (2.0581, 25.0004) -> (3.2443, 25.0004)
  line L647 (3.2443, 25.0004) -> (6.8079, 24.7632)
  line L648 (6.8079, 24.7632) -> (11.4231, 24.0672)
  line L649 (11.4231, 24.0672) -> (15.8783, 22.9344)
  line L650 (15.8783, 22.9344) -> (20.1506, 21.3883)
  line L651 (20.1506, 21.3883) -> (24.2146, 19.4535)
  line L652 (24.2146, 19.4535) -> (28.0449, 17.151)
  line L653 (28.0449, 17.151) -> (31.6237, 14.5051)
  line L654 (31.6237, 14.5051) -> (34.9257, 11.5384)
  line L655 (34.9257, 11.5384) -> (37.9255, 8.2752)
  line L656 (37.9255, 8.2752) -> (40.6026, 4.736)
  line L657 (40.6026, 4.736) -> (42.9293, 0.9466)
  line L658 (42.9293, 0.9466) -> (44.8876, -3.0704)
  line L659 (44.8876, -3.0704) -> (46.4497, -7.2927)
  line L660 (46.4497, -7.2927) -> (47.5953, -11.6983)
  line L661 (47.5953, -11.6983) -> (48.2988, -16.2609)
  line L662 (48.2988, -16.2609) -> (48.5401, -19.7859)
  line L663 (48.5401, -19.7859) -> (48.5401, -20.9614)
  line L664 (-45.114, 13.021) -> (-45.114, 12.5442)
  line L665 (-45.114, 12.5442) -> (-45.3098, 11.1124)
  line L666 (-45.3098, 11.1124) -> (-45.8681, 9.3334)
  line L667 (-45.8681, 9.3334) -> (-46.7513, 7.7238)
  line L668 (-46.7513, 7.7238) -> (-47.9212, 6.3222)
  line L669 (-47.9212, 6.3222) -> (-49.339, 5.1648)
  line L670 (-49.339, 5.1648) -> (-50.9682, 4.2913)
  line L671 (-50.9682, 4.2913) -> (-52.7662, 3.7386)
  line L672 (-52.7662, 3.7386) -> (-54.2148, 3.5455)
  line L673 (-54.2148, 3.5455) -> (-54.6969, 3.5455)
  line L674 (-54.6969, 3.5455) -> (-55.1805, 3.5455)
  line L675 (-55.1805, 3.5455) -> (-56.6291, 3.7386)
  line L676 (-56.6291, 3.7386) -> (-58.4287, 4.2913)
  line L677 (-58.4287, 4.2913) -> (-60.056, 5.1648)
  line L678 (-60.056, 5.1648) -> (-61.4741, 6.3222)
  line L679 (-61.4741, 6.3222) -> (-62.6453, 7.7238)
  line L680 (-62.6453, 7.7238) -> (-63.5287, 9.3334)
  line L681 (-63.5287, 9.3334) -> (-64.0868, 11.1124)
  line L682 (-64.0868, 11.1124) -> (-64.2813, 12.5442)
  line L683 (-64.2813, 12.5442) -> (-64.2813, 13.021)
  line L684 (-64.2813, 13.021) -> (-64.2813, 13.499)
  line L685 (-64.2813, 13.499) -> (-64.0868, 14.9311)
  line L686 (-64.0868, 14.9311) -> (-63.5287, 16.7101)
  line L687 (-63.5287, 16.7101) -> (-62.6453, 18.3194)
  line L688 (-62.6453, 18.3194) -> (-61.4741, 19.7225)
  line L689 (-61.4741, 19.7225) -> (-60.056, 20.88)
  line L690 (-60.056, 20.88) -> (-58.4287, 21.7538)
  line L691 (-58.4287, 21.7538) -> (-56.6291, 22.3062)
  line L692 (-56.6291, 22.3062) -> (-55.1805, 22.4977)
  line L693 (-55.1805, 22.4977) -> (-54.6969, 22.4977)
  line L694 (-54.6969, 22.4977) -> (-54.2148, 22.4977)
  line L695 (-54.2148, 22.4977) -> (-52.7662, 22.3062)
  line L696 (-52.7662, 22.3062) -> (-50.9682, 21.7538)
  line L697 (-50.9682, 21.7538) -> (-49.339, 20.88)
  line L698 (-49.339, 20.88) -> (-47.9212, 19.7225)
  line L699 (-47.9212, 19.7225) -> (-46.7513, 18.3194)
  line L700 (-46.7513, 18.3194) -> (-45.8681, 16.7101)
  line L701 (-45.8681, 16.7101) -> (-45.3098, 14.9311)
  line L702 (-45.3098, 14.9311) -> (-45.114, 13.499)
  line L703 (-45.114, 13.499) -> (-45.114, 13.021)
  line L704 (-44.7337, -54.9426) -> (-44.7337, -55.4193)
  line L705 (-44.7337, -55.4193) -> (-44.9293, -56.8511)
  line L706 (-44.9293, -56.8511) -> (-45.4876, -58.6301)
  line L707 (-45.4876, -58.6301) -> (-46.3708, -60.2395)
  line L708 (-46.3708, -60.2395) -> (-47.541, -61.6426)
  line L709 (-47.541, -61.6426) -> (-48.9588, -62.8)
  line L710 (-48.9588, -62.8) -> (-50.5877, -63.6738)
  line L711 (-50.5877, -63.6738) -> (-52.386, -64.2263)
  line L712 (-52.386, -64.2263) -> (-53.8343, -64.4193)
  line L713 (-53.8343, -64.4193) -> (-54.3167, -64.4193)
  line L714 (-54.3167, -64.4193) -> (-54.8003, -64.4193)
  line L715 (-54.8003, -64.4193) -> (-56.2486, -64.2263)
  line L716 (-56.2486, -64.2263) -> (-58.0484, -63.6738)
  line L717 (-58.0484, -63.6738) -> (-59.6758, -62.8)
  line L718 (-59.6758, -62.8) -> (-61.0939, -61.6426)
  line L719 (-61.0939, -61.6426) -> (-62.2651, -60.2395)
  line L720 (-62.2651, -60.2395) -> (-63.1485, -58.6301)
  line L721 (-63.1485, -58.6301) -> (-63.7065, -56.8511)
  line L722 (-63.7065, -56.8511) -> (-63.9008, -55.4193)
  line L723 (-63.9008, -55.4193) -> (-63.9008, -54.9426)
  line L724 (-63.9008, -54.9426) -> (-63.9008, -54.4643)
  line L725 (-63.9008, -54.4643) -> (-63.7065, -53.0327)
  line L726 (-63.7065, -53.0327) -> (-63.1485, -51.2537)
  line L727 (-63.1485, -51.2537) -> (-62.2651, -49.6439)
  line L728 (-62.2651, -49.6439) -> (-61.0939, -48.2413)
  line L729 (-61.0939, -48.2413) -> (-59.6758, -47.0848)
  line L730 (-59.6758, -47.0848) -> (-58.0484, -46.2113)
  line L731 (-58.0484, -46.2113) -> (-56.2486, -45.6586)
  line L732 (-56.2486, -45.6586) -> (-54.8003, -45.4671)
  line L733 (-54.8003, -45.4671) -> (-54.3167, -45.4671)
  line L734 (-54.3167, -45.4671) -> (-53.8343, -45.4671)
  line L735 (-53.8343, -45.4671) -> (-52.386, -45.6586)
  line L736 (-52.386, -45.6586) -> (-50.5877, -46.2113)
  line L737 (-50.5877, -46.2113) -> (-48.9588, -47.0848)
  line L738 (-48.9588, -47.0848) -> (-47.541, -48.2413)
  line L739 (-47.541, -48.2413) -> (-46.3708, -49.6439)
  line L740 (-46.3708, -49.6439) -> (-45.4876, -51.2537)
  line L741 (-45.4876, -51.2537) -> (-44.9293, -53.0327)
  line L742 (-44.9293, -53.0327) -> (-44.7337, -54.4643)
  line L743 (-44.7337, -54.4643) -> (-44.7337, -54.9426)
  point P0 (-62.6878, 18.2421)
  point P1 (-46.7088, 18.2421)
  point P2 (-143.5852, 12.9744)
  point P3 (-65.4262, -26.2772)
  point P4 (-98.6427, -70.4071)
  point P5 (-61.6859, -70.4071)
  point P6 (-62.9714, -58.9527)
  point P7 (-45.6482, -58.9227)
  point P8 (-46.9172, -70.4071)
  point P9 (-12.9827, -70.4071)
  point P10 (-43.9721, -27.042)
  point P11 (34.4002, 12.0106)
  point P12 (-7.0451, -72.2478)
  point P13 (-49.19, -72.2478)
  point P14 (-59.4125, -72.2478)
  point P15 (-106.4631, -72.2478)
  point P16 (48.9777, -44.8768)
  point P17 (-155.8218, -48.991)
  point P18 (-147.4018, -55.7632)
  point P19 (-131.5571, 25.3247)
  point P20 (48.7072, -1.2292)
  point P21 (48.7037, -39.9263)
  constraints: 1488 end point
extrude "Extrusion21" add sketch "Sketch1" along normal blind 0.25 contours L15 L16 L17 L18 L19 L20 L21 L22 L23 L24 L25 L26 L27 L28 L29 L309 L308 L307 L306 L305 L304 L303 L302 L301 L300 L299 L298 | L298 L190 L191 L192 L193 L194 L195 L196 L197 | L298 L371 L370 L369 L368 L367 L366 L365 L364 L363 L362 L361 L360 L77 L78 L79 L80 L81 L82 L83 L84 L85 L86 L87 L88 L89 L90 L91 L92 L93 | L224 L225 L226 L227 L228 L229 L230 L231 L232 L233 L234 L235 L236 L237 L238 L239 L240 L241 L242 L243 L244 L245 L246 L247 L248 L249 L250 L251 L252 L253 L254 L255 L256 L257 L258 L259 L260 L261 L262 L263 L264 L265 L266 L267 L268 L269 L270 L271 L272 L273 L274 L275 L276 L277 L278 L279 L280 L281 L282 L283 L284 L285 L286 L287 L288 L289 L290 L291 L292 L293 L294 L295 L296 L297
extrude "Extrusion22" add sketch "Sketch1" along normal blind 0.5 contours L372 L199 L198 L197 L298 L15 L14 L13 | L13 L14 L15 L298 L299 L300 L301 L302 L303 L304 L305 L306 L307 L308 L309 L29 L30 L31 L32 L33 L34 L35 L36 L37 L38 L392 L391 L390 L389 L388 L387 L386 L385 L384 L383 L382 L381 L380 L379 L378 L377 L376 L375 L374 L373 L372 | L372 L188 L189 L190 L298 L197 L198 L199 | L372 L94 L93 L298 L190 L189 L188 | L372 L445 L444 L443 L442 L441 L440 L439 L438 L437 L436 L435 L434 L433 L432 L431 L430 L429 L428 L427 L141 L142 L143 L72 L73 L74 L75 L76 L77 L360 L361 L362 L363 L364 L365 L366 L367 L368 L369 L370 L371 L298 L93 L94 | L309 L310 L311 L312 L313 L314 L315 L316 L317 L318 L319 L320 L321 L322 L323 L324 L325 L326 L327 L328 L329 L330 L331 L332 L333 L334 L335 L336 L337 L338 L339 L340 L341 L342 L343 L344 L345 L346 L347 L348 L349 L350 L351 L352 L353 L354 L355 L356 L357 L358 L359 L360 L77 L76 L75 L74 L73 L72 L143 L142 L141 L427 L426 L425 L424 L423 L422 L421 L420 L419 L418 L417 L416 L415 L414 L413 L412 L411 L410 L409 L408 L407 L406 L405 L404 L403 L402 L401 L400 L399 L398 L397 L396 L395 L394 L393 L392 L38 L37 L36 L35 L34 L33 L32 L31 L30 L29
extrude "Extrusion23" add sketch "Sketch1" along normal blind 0.25 contours L71 L70 L69 L68 L67 L66 L65 L64 L63 L62 L61 L60 L59 L58 L57 L56 L55 L54 L53 L52 L51 L50 L49 L48 L47 L46 L565 L566 L567 L568 L569 L570 L571 L572 L573 L574 L575 L576 L577 L578 L579 L580 L581 L582 L583 L584 L585 L586 L587 L588 L589 L590 L591 L520 L521 L522 L1 L0 | L0 L1 L522 L523 L524 L525 L526 L527 L528 L529 L530 L531 L532 L533 L534 L535 L536 L537 L538 L539 L540 L541 L542 L543 L544 L545 L546 L547 L548 L549 L550 L551 L552 L553 L554 L555 L556 L557 L558 L559 L560 L561 L562 L563 L564 L565 L46 L47 L48 L49 L50 L51 L52 L53 L54 L55 L56 L57 L58 L59 L60 L61 L62 L63 L64 L65 L66 L67 L68 L69 L70 L71 | L522 L521 L520 L591 L590 L589 L588 L587 L586 L585 L584 L583 L582 L581 L580 L579 L578 L577 L576 L575 L574 L573 L572 L571 L570 L569 L568 L567 L566 L565 L46 L45 L44 L43 L42 L41 L40 L39 L38 L392 L393 L394 L395 L396 L397 L398 L399 L400 L401 L402 L403 L404 L405 L406 L407 L408 L409 L410 L411 L412 L413 L414 L415 L416 L417 L418 L419 L420 L421 L422 L423 L424 L425 L426 L427 L141 L140 L139 L138 L137 L136 L135 L134 L133 L654 L653 L652 L651 L650 L649 L648 L647 L646 L645 L644 L643 L642 L641 L640 L639 L638 L637 L636 L635 L634 L633 L632 L631 L630 L629 L628 L627 L626 L625 L106 L105 L104 L103 L102 L101 L100 L99 L98 L97 L96 L95 L94 L372 L188 L187 L186 L185 L184 L223 L222 L221 L220 L707 L706 L705 L704 L743 L742 L741 L740 L739 L738 L737 L736 L735 L734 L733 L732 L731 L730 L729 L728 L727 L726 L725 L724 L723 L722 L721 L720 L207 L206 L205 L204 L203 L202 L201 L200 L199 L13 L12 L11 L10 L9 L8 L7 L6 L5 L4 L3 L2 L1 | L1 L2 L3 L4 L5 L6 L7 L8 L9 L10 L11 L12 L13 L372 L373 L374 L375 L376 L377 L378 L379 L380 L381 L382 L383 L384 L385 L386 L387 L388 L389 L390 L391 L392 L38 L39 L40 L41 L42 L43 L44 L45 L46 L565 L564 L563 L562 L561 L560 L559 L558 L557 L556 L555 L554 L553 L552 L551 L550 L549 L548 L547 L546 L545 L544 L543 L542 L541 L540 L539 L538 L537 L536 L535 L534 L533 L532 L531 L530 L529 L528 L527 L526 L525 L524 L523 L522 | L199 L200 L201 L202 L203 L204 L205 L206 L207 L720 L719 L718 L717 L716 L715 L714 L713 L712 L711 L710 L709 L708 L707 L220 L221 L222 L223 L184 L185 L186 L187 L188 L372 | L94 L95 L96 L97 L98 L99 L100 L101 L102 L103 L104 L105 L106 L625 L624 L623 L622 L621 L620 L619 L618 L617 L616 L615 L614 L613 L612 L611 L610 L609 L608 L607 L606 L605 L604 L603 L602 L601 L600 L599 L598 L597 L596 L595 L594 L593 L592 L663 L662 L661 L660 L659 L658 L657 L656 L655 L654 L133 L134 L135 L136 L137 L138 L139 L140 L141 L427 L428 L429 L430 L431 L432 L433 L434 L435 L436 L437 L438 L439 L440 L441 L442 L443 L444 L445 L372 | L720 L721 L722 L723 L724 L725 L726 L727 L728 L729 L730 L731 L732 L733 L734 L735 L736 L737 L738 L739 L740 L741 L742 L743 L704 L705 L706 L707 L220 L219 L218 L217 L216 L215 L214 L213 L212 L211 L210 L209 L208 L207 | L207 L208 L209 L210 L211 L212 L213 L214 L215 L216 L217 L218 L219 L220 L707 L708 L709 L710 L711 L712 L713 L714 L715 L716 L717 L718 L719 L720 | L625 L626 L627 L628 L629 L630 L631 L632 L633 L634 L635 L636 L637 L638 L639 L640 L641 L642 L643 L644 L645 L646 L647 L648 L649 L650 L651 L652 L653 L654 L133 L132 L131 L130 L129 L128 L127 L126 L125 L124 L123 L122 L121 L120 L119 L118 L117 L116 L115 L114 L113 L112 L111 L110 L109 L108 L107 L106 | L106 L107 L108 L109 L110 L111 L112 L113 L114 L115 L116 L117 L118 L119 L120 L121 L122 L123 L124 L125 L126 L127 L128 L129 L130 L131 L132 L133 L654 L655 L656 L657 L658 L659 L660 L661 L662 L663 L592 L593 L594 L595 L596 L597 L598 L599 L600 L601 L602 L603 L604 L605 L606 L607 L608 L609 L610 L611 L612 L613 L614 L615 L616 L617 L618 L619 L620 L621 L622 L623 L624 L625 | L144 L145 L146 L147 L148 L149 L150 L151 L152 L153 L154 L155 L156 L157 L158 L159 L160 L161 L162 L163 L164 L165 L166 L167 L168 L687 L686 L685 L684 L683 L682 L681 L680 L679 L678 L677 L676 L675 L674 L673 L672 L671 L670 L669 L668 L667 L666 L665 L664 L703 L702 L701 L700 L179 L180 L181 L182 L183 | L700 L701 L702 L703 L664 L665 L666 L667 L668 L669 L670 L671 L672 L673 L674 L675 L676 L677 L678 L679 L680 L681 L682 L683 L684 L685 L686 L687 L168 L169 L170 L171 L172 L173 L174 L175 L176 L177 L178 L179 | L179 L178 L177 L176 L175 L174 L173 L172 L171 L170 L169 L168 L687 L688 L689 L690 L691 L692 L693 L694 L695 L696 L697 L698 L699 L700